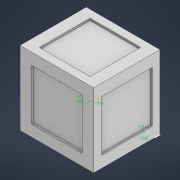
# Autodesk Inventor part: End-Effector
Saved by Autodesk Inventor 2022 (Build 260153000, 153)
## iProperties
Created: 2023-04-20
Part Number: End-Effector
Material: Generic
Document SubType Name: Modeling
Designer: Karl
Density: 1 g/cm^3
Appearance: Default
Author: Karl
Autodesk Inventor part; units mm, degrees
ref_plane "YZ Plane" through (0, 0, 0) normal (1, 0, 0) x (0, 1, 0)
ref_plane "XZ Plane" through (0, 0, 0) normal (0, 1, 0) x (-1, 0, 0)
ref_plane "XY Plane" through (0, 0, 0) normal (0, 0, 1) x (1, 0, 0)
sketch "Sketch3" plane through (0, 0, 0) normal (0, 0, 1) x (1, 0, 0)
  line L0 (0, 0) -> (-80, 0)
  line L1 (-80, 0) -> (-80, 80)
  line L2 (-80, 80) -> (0, 80)
  line L3 (0, 80) -> (0, 0)
  line L4 (-75, 75) -> (-5, 75)
  line L5 (-5, 75) -> (-5, 5)
  line L6 (-5, 5) -> (-75, 5)
  line L7 (-75, 5) -> (-75, 75)
  dimension "d129" = 80
  dimension "d130" = 80
  dimension "d131" = 70
  dimension "d132" = 70
  constraints: 16 end point, 4 parallel, 2 horizontal, 2 perpendicular
  measures "d129" distance of L1.end L2.end
  measures "d130" distance of L0.end L1.end
  measures "d131" distance of L5.end L6.end
  measures "d132" distance of L4.end L5.end
extrude "Extrusion19" add sketch "Sketch3" along normal blind 68
sketch "Sketch18" plane through (0, 0, 68) normal (0, 0, 1) x (1, 0, 0)
  line L0 (0, 80) -> (-80, 80) projected
  line L1 (0, 0) -> (-80, 0)
  line L2 (-80, 0) -> (-80, 80)
  line L3 (-80, 80) -> (0, 80)
  line L4 (0, 80) -> (0, 0)
  dimension "d135" = 80
  dimension "d136" = 80
  constraints: 8 end point, 2 parallel, 1 horizontal, 1 perpendicular
  measures "d135" distance of L0.end L3.end
  measures "d136" distance of L1.end L0.end
extrude "Extrusion20" add sketch "Sketch18" along normal blind 4
sketch "Sketch20" plane through (0, 0, 72) normal (0, 0, 1) x (1, 0, 0)
  line L0 (-67.5, 67.5) -> (-12.5, 67.5)
  line L1 (-12.5, 67.5) -> (-12.5, 12.5)
  line L2 (-12.5, 12.5) -> (-67.5, 12.5)
  line L3 (-67.5, 12.5) -> (-67.5, 67.5)
  point P0 (0, 0)
  dimension "d139" = 55
  dimension "d140" = 55
  constraints: 8 end point, 2 parallel, 1 horizontal, 1 perpendicular
  measures "d139" distance of L1.end L2.end
  measures "d140" distance of L0.end L1.end
extrude "Extrusion21" cut sketch "Sketch20" against normal blind 2
sketch "Sketch21" plane through (0, 0, 0) normal (1, 0, 0) x (0, 0, -1)
  line L0 (-63.5, 12.5) -> (-8.5, 12.5)
  line L1 (-8.5, 12.5) -> (-8.5, 67.5)
  line L2 (-8.5, 67.5) -> (-63.5, 67.5)
  line L3 (-63.5, 67.5) -> (-63.5, 12.5)
  point P0 (0, 0)
  dimension "d143" = 55
  dimension "d144" = 55
  constraints: 8 end point, 2 parallel, 1 horizontal, 1 perpendicular
  measures "d143" distance of L2.end L1.end
  measures "d144" distance of L1.end L0.end
sketch "Sketch22" plane through (-80, 0, 0) normal (-1, 0, 0) x (0, 0, 1)
  line L0 (8.5, 12.5) -> (63.5, 12.5)
  line L1 (63.5, 12.5) -> (63.5, 67.5)
  line L2 (63.5, 67.5) -> (8.5, 67.5)
  line L3 (8.5, 67.5) -> (8.5, 12.5)
  point P0 (0, 0)
  dimension "d145" = 55
  dimension "d146" = 55
  constraints: 8 end point, 2 parallel, 1 horizontal, 1 perpendicular
  measures "d145" distance of L2.end L1.end
  measures "d146" distance of L1.end L0.end
sketch "Sketch23" plane through (-80, 0, 0) normal (0, -1, 0) x (1, 0, 0)
  line L0 (12.5, 8.5) -> (67.5, 8.5)
  line L1 (67.5, 8.5) -> (67.5, 63.5)
  line L2 (67.5, 63.5) -> (12.5, 63.5)
  line L3 (12.5, 63.5) -> (12.5, 8.5)
  point P0 (80, 0)
  dimension "d147" = 55
  dimension "d148" = 55
  constraints: 8 end point, 2 parallel, 1 horizontal, 1 perpendicular
  measures "d147" distance of L2.end L1.end
  measures "d148" distance of L1.end L0.end
sketch "Sketch24" plane through (-80, 80, 0) normal (0, 1, 0) x (1, 0, 0)
  line L0 (12.5, -8.5) -> (67.5, -8.5)
  line L1 (67.5, -8.5) -> (67.5, -63.5)
  line L2 (67.5, -63.5) -> (12.5, -63.5)
  line L3 (12.5, -63.5) -> (12.5, -8.5)
  point P0 (80, 0)
  dimension "d149" = 55
  dimension "d150" = 55
  constraints: 8 end point, 2 parallel, 1 horizontal, 1 perpendicular
  measures "d149" distance of L1.end L2.end
  measures "d150" distance of L0.end L1.end
extrude "Extrusion22" cut sketch "Sketch21" against normal blind 2
extrude "Extrusion23" cut sketch "Sketch24" against normal blind 2
extrude "Extrusion24" cut sketch "Sketch23" against normal blind 2
extrude "Extrusion25" cut sketch "Sketch22" against normal blind 2
sketch "Sketch25" plane through (-80, 0, 0) normal (0, -1, 0) x (1, 0, 0)
  line L0 (80, 0) -> (0, 0) projected
  line L1 (0, 0) -> (10.6, 0)
  line L2 (10.6, 0) -> (10.6, 5.6)
  line L3 (10.6, 5.6) -> (0, 5.6)
  line L4 (0, 5.6) -> (0, 0)
  line L5 (80, 0) -> (69.4, 0)
  line L6 (69.4, 0) -> (69.4, 5.6)
  line L7 (69.4, 5.6) -> (80, 5.6)
  line L8 (80, 5.6) -> (80, 0)
  dimension "d159" = 10.6
  dimension "d160" = 5.6
  dimension "d161" = 10.6
  dimension "d162" = 5.6
  constraints: 16 end point, 4 parallel, 2 horizontal, 2 perpendicular
  measures "d159" distance of L3.end L2.end
  measures "d160" distance of L2.end L1.end
  measures "d161" distance of L6.end L7.end
  measures "d162" distance of L5.end L6.end
body "Solid4"
